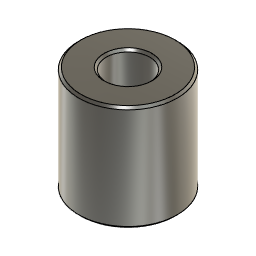
ShooterSpacer (Autodesk Fusion 360 design; units mm, degrees)
Autodesk Fusion 360 part; units mm, degrees
sketch "Sketch1" plane through (0, 0, 0) normal (0, 0, 1) x (1, 0, 0)
  circle A0 centre (0, 0) radius 7.95
  circle A1 centre (0, 0) radius 3.5
  dimension "d1" = 15.9
  dimension "d2" = 7
  constraint coincident A0.centre A1.centre
  constraint concentric A0 A1
  measures "d1" diameter of A0
  measures "d2" diameter of A1
extrude "Extrude1" add sketch "Sketch1" along normal blind 17
chamfer "Chamfer1" distance 0.35 angle 45 4 edges at (-3.2631, 1.2657, 17) (-3.2631, 1.2657, 0) (-7.412, -2.8748, 0) (-7.412, -2.8748, 17)
